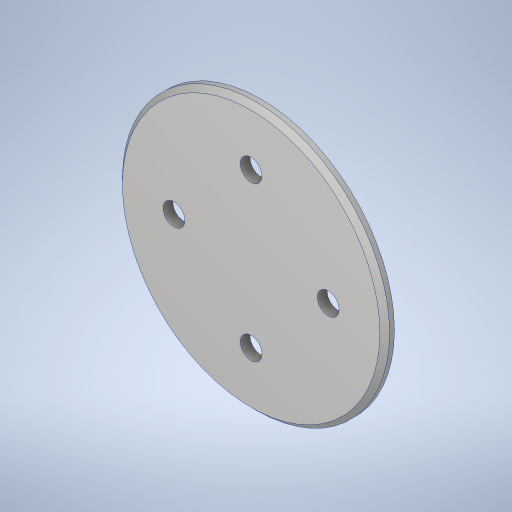
# Autodesk Inventor part: 53t_gt2_flange
Saved by Autodesk Inventor 2023.3 (Build 273359000, 359)
## iProperties
Created: 2024-02-17
Part Number: 53t_gt2_flange
Material: Aluminum 6061
Document SubType Name: Modeling
Designer: mavericks
Density: 2.7 g/cm^3
Appearance: Aluminum - Flat
Author: mavericks
Autodesk Inventor part; units mm, degrees
ref_plane "YZ Plane" through (0, 0, 0) normal (1, 0, 0) x (0, 1, 0)
ref_plane "XZ Plane" through (0, 0, 0) normal (0, 1, 0) x (-1, 0, 0)
ref_plane "XY Plane" through (0, 0, 0) normal (0, 0, 1) x (1, 0, 0)
sketch "Sketch1" plane through (0, 0, 0) normal (0, 0, 1) x (1, 0, 0)
  circle A0 centre (0, 0) radius 27.5
  dimension "d0" = 55
  constraints: 1 centre point, 1 coincident
  measures "d0" diameter of A0
extrude "Extrusion1" add sketch "Sketch1" along normal blind 2
chamfer "Chamfer1" distance 1 angle 45 1 edges at (-27.5, 0, 2)
sketch "Sketch2" plane through (0, 0, 2) normal (0, 0, 1) x (1, 0, 0)
  circle A0 centre (0, 0) radius 15.875 construction
  point P0 (0, 15.875)
  point P1 (-15.875, 0)
  point P2 (0, -15.875)
  point P3 (15.875, 0)
  dimension "d6" = 31.75
  dimension "d9" = 360
  constraints: 1 coincident, 1 vertical alignment, 7 other
hole "Hole1" at (0, 15.875, 2) at (-15.875, 0, 2) at (0, -15.875, 2) at (15.875, 0, 2) direction (0, 0, -1) diameter 4.4958 end through all clearance for "Flat Head Machine Screw (82)" size "#8" standard "Ansi Unified Screw Threads"
body "Solid1"
